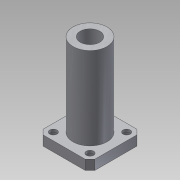
# Autodesk Inventor part: Z-flange
Saved by Autodesk Inventor 2016 (Build 200138000, 138)
## iProperties
Created: 2015-06-08
Part Number: Z-flange
Material: Aluminum 6061
Document SubType Name: Modeling
Designer: Mathias L. Kjeldgaard
Density: 2.71 g/cm^3
Appearance: Aluminum - Flat
Mass: 44.0846 g
Surface Area: 84.307 cm^2
Volume: 16.2674 cm^3
Author: Mathias L. Kjeldgaard
Autodesk Inventor part; units mm, degrees
ref_plane "YZ Plane" through (0, 0, 0) normal (1, 0, 0) x (0, 1, 0)
ref_plane "XZ Plane" through (0, 0, 0) normal (0, 1, 0) x (-1, 0, 0)
ref_plane "XY Plane" through (0, 0, 0) normal (0, 0, 1) x (1, 0, 0)
sketch "Sketch1" plane through (0, 0, 0) normal (0, 0, 1) x (1, 0, 0)
  line L0 (-16, 16) -> (16, 16)
  line L1 (16, 16) -> (16, -16)
  line L2 (16, -16) -> (-16, -16)
  line L3 (-16, -16) -> (-16, 16)
  point P0 (0, 0)
  dimension "d0" = 32
  dimension "d1" = 32
  dimension "d2" = 16
  dimension "d3" = 16
  constraints: 8 end point, 2 parallel, 1 horizontal, 1 perpendicular
  measures "d0" distance of L1.end L2.end
  measures "d1" distance of L0.end L1.end
  measures "d2" distance from line of L1 point (0, 0)
  measures "d3" distance from line of L0 point (0, 0)
extrude "Firkant" add sketch "Sketch1" along normal blind 6
sketch "Sketch2" plane through (0, 0, 6) normal (0, 0, 1) x (1, 0, 0)
  circle A0 centre (0, 0) radius 10.5
  dimension "d6" = 21
  constraints: 1 centre point, 1 coincident
  measures "d6" diameter of A0
extrude "Rør" add sketch "Sketch2" along normal blind 51
sketch "Sketch3" plane through (0, 0, 0) normal (0, 0, -1) x (-1, 0, 0)
  circle A0 centre (0, 0) radius 6
  dimension "d9" = 12
  constraints: 1 centre point, 1 coincident
  measures "d9" diameter of A0
extrude "Hul" cut sketch "Sketch3" against normal up to surface (57 mm away)
sketch "Sketch4" plane through (0, 0, 6) normal (0, 0, 1) x (1, 0, 0)
  circle A0 centre (0, 0) radius 10.5 construction
  circle A1 centre (0, 0) radius 16 construction
  line L0 (-16, 16) -> (16, -16) construction
  line L1 (16, 16) -> (-16, -16) construction
  circle A2 centre (11.3137, 11.3137) radius 2.25
  circle A3 centre (-11.3137, 11.3137) radius 2.25
  circle A4 centre (-11.3137, -11.3137) radius 2.25
  circle A5 centre (11.3137, -11.3137) radius 2.25
  dimension "d12" = 32
  dimension "d13" = 4.5
  dimension "d14" = 4.5
  dimension "d15" = 4.5
  dimension "d16" = 4.5
  constraints: 5 centre point, 4 end point, 4 point on circle, 4 point on line, 1 coincident, 1 perpendicular
  measures "d12" diameter of A1
  measures "d13" diameter of A5
  measures "d14" diameter of A2
  measures "d15" diameter of A3
  measures "d16" diameter of A4
extrude "d1 Hullerne (små)" cut sketch "Sketch4" against normal up to surface (6 mm away)
sketch "Sketch5" plane through (0, 0, 0) normal (0, 0, -1) x (-1, 0, 0)
  circle A0 centre (11.3137, -11.3137) radius 2.25 projected
  circle A1 centre (-11.3137, -11.3137) radius 2.25 projected
  circle A2 centre (11.3137, 11.3137) radius 2.25 projected
  circle A3 centre (-11.3137, 11.3137) radius 2.25 projected
  circle A4 centre (-11.3137, 11.3137) radius 4
  circle A5 centre (11.3137, 11.3137) radius 4
  circle A6 centre (11.3137, -11.3137) radius 4
  circle A7 centre (-11.3137, -11.3137) radius 4
  dimension "d19" = 8
  dimension "d20" = 8
  dimension "d21" = 8
  dimension "d22" = 8
  constraints: 4 centre point, 4 coincident
  measures "d19" diameter of A6
  measures "d20" diameter of A5
  measures "d21" diameter of A4
  measures "d22" diameter of A7
extrude "d2 Hullerne (store)" cut sketch "Sketch5" against normal blind 4.4
chamfer "Hjørnerne" distance 3 angle 45 4 edges at (-16, -16, 3) (16, -16, 3) (16, 16, 3) (-16, 16, 3)
equation "\"d1\" = d0"
equation "\"d2\" = 0.5 * d0"
equation "\"d3\" = 0.5 * d1"
equation "\"d14\" = d13"
equation "\"d15\" = d13"
equation "\"d16\" = d13"
equation "\"d20\" = d19"
equation "\"d21\" = d19"
equation "\"d22\" = d19"
body "Solid1"
